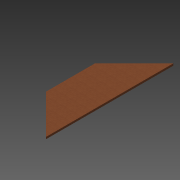
# Autodesk Inventor part: top short
Saved by Autodesk Inventor 2015 (Build 190159000, 159)
## iProperties
Created: 2019-04-10
Part Number: top short
Material: Generic
Document SubType Name: Modeling
Designer: Raptor
Density: 1 g/cm^3
Appearance: English Oak
Author: Raptor
Autodesk Inventor part; units mm, degrees
ref_plane "YZ Plane" through (0, 0, 0) normal (1, 0, 0) x (0, 1, 0)
ref_plane "XZ Plane" through (0, 0, 0) normal (0, 1, 0) x (-1, 0, 0)
ref_plane "XY Plane" through (0, 0, 0) normal (0, 0, 1) x (1, 0, 0)
sketch "Sketch1" plane through (0, 0, 0) normal (0, 1, 0) x (-1, 0, 0)
  line L0 (0, 0) -> (0, -1300)
  line L1 (0, -1300) -> (400, -900)
  line L2 (400, -900) -> (400, -400)
  line L3 (0, 0) -> (400, -400)
  dimension "d0" = 45
  dimension "d1" = 45
  dimension "d2" = 500
  dimension "d3" = 1300
  constraints: 8 end point, 1 parallel, 1 vertical
  measures "d0" angle of L0 L3
  measures "d1" angle of L1 L0
  measures "d2" distance of L1.end L2.end
  measures "d3" distance of L0.start L0.end
extrude "Extrusion1" add sketch "Sketch1" along normal blind 20
body "Solid1"
